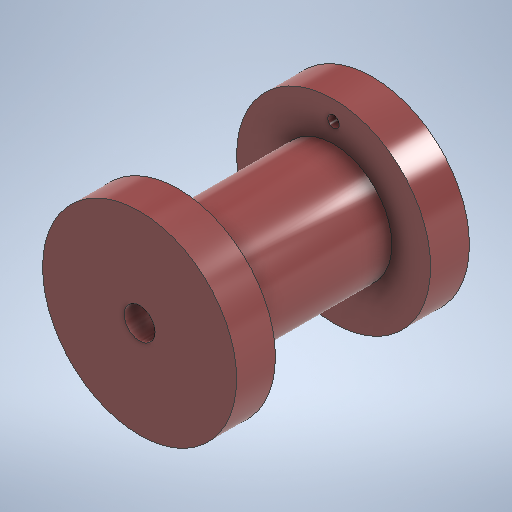
# Autodesk Inventor part: carrete
Saved by Autodesk Inventor 2026 (Build 300175050, 175E)
## iProperties
Created: 2025-06-24
Part Number: carrete
Material: Genérico
Document SubType Name: Modeling
Designer: piero
Density: 1 g/cm^3
Appearance: Valor por defecto
Author: piero
Autodesk Inventor part; units mm, degrees
ref_plane "YZ Plane" through (0, 0, 0) normal (1, 0, 0) x (0, 1, 0)
ref_plane "XZ Plane" through (0, 0, 0) normal (0, 1, 0) x (-1, 0, 0)
ref_plane "XY Plane" through (0, 0, 0) normal (0, 0, 1) x (1, 0, 0)
sketch "Boceto1" plane through (0, 0, 0) normal (0, 0, 1) x (1, 0, 0)
  circle A0 centre (0, 0) radius 25
  circle A1 centre (0, 0) radius 4
  circle A2 centre (0, 0) radius 11
  dimension "d0" = 50
  dimension "d3" = 8
  dimension "d34" = 22
  constraints: 3 centre point, 3 coincident
  measures "d0" diameter of A0
  measures "d3" diameter of A1
  measures "d34" diameter of A2
extrude "Extrusión1" add sketch "Boceto1" along normal blind 10 contours A0 | A2
sketch "Boceto5" plane through (0, 0, 10) normal (0, 0, 1) x (1, 0, 0)
  circle A0 centre (0, 0) radius 4
  circle A1 centre (0, 0) radius 15
  dimension "d15" = 8
  dimension "d16" = 30
  constraints: 2 centre point, 2 coincident
  measures "d15" diameter of A0
  measures "d16" diameter of A1
extrude "Extrusión5" add sketch "Boceto5" along normal blind 40
sketch "Boceto6" plane through (0, 0, 50) normal (0, 0, 1) x (1, 0, 0)
  circle A0 centre (0, 0) radius 4 projected
  circle A1 centre (0, 0) radius 25
  circle A2 centre (0, 0) radius 4
  circle A3 centre (0, 0) radius 11
  dimension "d22" = 50
  dimension "d30" = 8
  dimension "d31" = 22
  constraints: 3 centre point, 2 coincident
  measures "d22" diameter of A1
  measures "d30" diameter of A2
  measures "d31" diameter of A3
extrude "Extrusión13" add sketch "Boceto6" along normal blind 10 contours A1 | A3
sketch "Boceto17" plane through (0, 0, 10) normal (0, 0, 1) x (1, 0, 0)
  circle A0 centre (0, 20.0085) radius 1.5
  point P0 (0, 0)
  dimension "d102" = 3
  constraints: 1 centre point
  measures "d102" diameter of A0
extrude "Extrusión14" cut sketch "Boceto17" against normal blind 10
